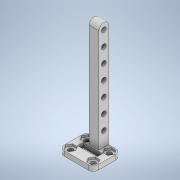
# Autodesk Inventor part: camera_stand
Saved by Autodesk Inventor 2020 (Build 240168000, 168)
## iProperties
Created: 2023-05-28
Part Number: camera_stand
Material: Generic
Document SubType Name: Modeling
Designer: denis
Density: 1 g/cm^3
Appearance: Default
Author: denis
Autodesk Inventor part; units mm, degrees
ref_plane "YZ Plane" through (0, 0, 0) normal (1, 0, 0) x (0, 1, 0)
ref_plane "XZ Plane" through (0, 0, 0) normal (0, 1, 0) x (-1, 0, 0)
ref_plane "XY Plane" through (0, 0, 0) normal (0, 0, 1) x (1, 0, 0)
sketch "Эскиз1" plane through (0, 0, 0) normal (1, 0, 0) x (0, 1, 0)
  line L0 (-2.5, 8.5) -> (0.5, 8.5)
  line L1 (0.5, 8.5) -> (0.5, -8.5)
  line L2 (0.5, -8.5) -> (-2.5, -8.5)
  line L3 (-2.5, -8.5) -> (-2.5, 8.5)
  line L4 (0.5, -8.5) -> (64.5, -8.5)
  line L5 (67.5, -5.5) -> (67.5, -5.5)
  line L6 (64.5, -2.5) -> (0.5, -2.5)
  line L7 (0.5, -2.5) -> (0.5, -8.5)
  circle A0 centre (9.5, -5.5) radius 1.5
  circle A1 centre (18.5, -5.5) radius 1.5
  circle A2 centre (27.5, -5.5) radius 1.5
  circle A3 centre (36.5, -5.5) radius 1.5
  circle A4 centre (45.5, -5.5) radius 1.5
  circle A5 centre (54.5, -5.5) radius 1.5
  circle A6 centre (63.5, -5.5) radius 1.5
  arc A7 (67.5, -5.5) -> (64.5, -2.5) centre (64.5, -5.5) ccw
  arc A8 (64.5, -8.5) -> (67.5, -5.5) centre (64.5, -5.5) ccw
  point P0 (0, 0)
  point P1 (67.5, -2.5)
  point P2 (67.5, -8.5)
  dimension "d0" = 3
  dimension "d1" = 17
  dimension "d2" = 67
  dimension "d3" = 6
  dimension "d4" = 3
  dimension "d5" = 9
  dimension "d6" = 3
  dimension "d7" = 9
  dimension "d8" = 3
  dimension "d9" = 9
  dimension "d10" = 3
  dimension "d11" = 9
  dimension "d12" = 3
  dimension "d13" = 9
  dimension "d14" = 3
  dimension "d15" = 9
  dimension "d16" = 3
  dimension "d17" = 9
  dimension "d18" = 3
  constraints: 16 end point, 9 centre point, 4 parallel, 4 point on circle, 4 point on line, 4 tangent, 2 horizontal, 2 perpendicular, 1 concentric
  measures "d0" distance of L1.end L2.end
  measures "d1" distance of L0.end L1.end
  measures "d2" distance of L6.end point (67.5, -2.5)
  measures "d3" distance of point (67.5, -2.5) point (67.5, -8.5)
  measures "d4" diameter of A0
  measures "d5" distance from line of L1 A0.centre
  measures "d6" diameter of A1
  measures "d7" distance of A0.centre A1.centre
  measures "d8" diameter of A2
  measures "d9" distance of A1.centre A2.centre
  measures "d10" diameter of A3
  measures "d11" distance of A2.centre A3.centre
  measures "d12" diameter of A4
  measures "d13" distance of A4.centre A3.centre
  measures "d14" diameter of A5
  measures "d15" distance of A4.centre A5.centre
  measures "d16" diameter of A6
  measures "d17" distance of A5.centre A6.centre
  measures "d18" radius of A7
extrude "Выдавливание1" add sketch "Эскиз1" along normal mid plane 21 contours L0 L1 L2 L3
extrude "Выдавливание2" add sketch "Эскиз1" along normal mid plane 6 contours L6 A7 A8 L4 L1
sketch "Эскиз3" plane through (-10.5, 0.5, 8.5) normal (0, 1, 0) x (1, 0, 0)
  line L0 (21, 0) -> (0, 0) projected
  line L1 (10.5, 0) -> (10.5, 17) construction
  line L2 (0, 17) -> (21, 17) projected
  line L3 (0, 17) -> (0, 0) construction
  line L4 (21, 0) -> (21, 17) construction
  line L5 (0, 0) -> (21, 17) construction
  line L6 (21, 0) -> (0, 17) construction
  line L7 (0, 8.5) -> (21, 8.5) construction
  circle A0 centre (3.5, 3.5) radius 1.5
  circle A1 centre (3.5, 13.5) radius 1.5
  circle A2 centre (17.5, 3.5) radius 1.5
  circle A3 centre (17.5, 13.5) radius 1.5
  line L8 (18, 0) -> (3, 0) construction
  line L9 (0, 3) -> (0, 14) construction
  line L10 (3, 17) -> (18, 17) construction
  line L11 (21, 14) -> (21, 3) construction
  line L12 (21, 0) -> (0, 17) construction
  line L13 (0, 0) -> (21, 17) construction
  arc A4 (3, 17) -> (0, 14) centre (3, 14) ccw
  arc A5 (0, 3) -> (3, 0) centre (3, 3) ccw
  arc A6 (18, 0) -> (21, 3) centre (18, 3) ccw
  arc A7 (21, 14) -> (18, 17) centre (18, 14) ccw
  line L14 (21, 0) -> (0, 0) construction
  line L15 (0, 0) -> (0, 17) construction
  line L16 (0, 17) -> (21, 17) construction
  line L17 (21, 17) -> (21, 0) construction
  line L18 (21, 0) -> (0, 17) construction
  line L19 (0, 0) -> (21, 17) construction
  line L20 (3, 0) -> (0, 0)
  line L21 (0, 0) -> (0, 3)
  line L22 (0, 14) -> (0, 17)
  line L23 (3, 17) -> (0, 17)
  line L24 (18, 17) -> (21, 17)
  line L25 (21, 17) -> (21, 14)
  line L26 (21, 3) -> (21, 0)
  line L27 (21, 0) -> (18, 0)
  line L28 (16.5, 6.75) -> (4.5, 6.75)
  line L29 (4.5, 6.75) -> (4.5, 10.25)
  line L30 (4.5, 10.25) -> (16.5, 10.25)
  line L31 (16.5, 10.25) -> (16.5, 6.75)
  line L32 (16.5, 6.75) -> (4.5, 10.25) construction
  line L33 (4.5, 6.75) -> (16.5, 10.25) construction
  line L34 (17.5, 3.5) -> (17.5, 0.65) construction
  line L35 (17.5, 0.65) -> (17.5, 6.35) construction
  line L36 (17.5, 3.5) -> (14.4, 3.5) construction
  line L37 (14.4, 3.5) -> (20.6, 3.5) construction
  line L38 (15.95, 0.8153) -> (14.4, 3.5)
  line L39 (14.4, 3.5) -> (15.95, 6.1847)
  line L40 (15.95, 6.1847) -> (19.05, 6.1847)
  line L41 (19.05, 6.1847) -> (20.6, 3.5)
  line L42 (20.6, 3.5) -> (19.05, 0.8153)
  line L43 (19.05, 0.8153) -> (15.95, 0.8153)
  line L44 (15.95, 10.8153) -> (14.4, 13.5)
  line L45 (15.95, 16.1847) -> (14.4, 13.5)
  line L46 (15.95, 10.8153) -> (19.05, 10.8153)
  line L47 (19.05, 10.8153) -> (20.6, 13.5)
  line L48 (20.6, 13.5) -> (19.05, 16.1847)
  line L49 (19.05, 16.1847) -> (15.95, 16.1847)
  line L50 (1.95, 0.8153) -> (0.4, 3.5)
  line L51 (0.4, 3.5) -> (1.95, 6.1847)
  line L52 (1.95, 6.1847) -> (5.05, 6.1847)
  line L53 (5.05, 6.1847) -> (6.6, 3.5)
  line L54 (6.6, 3.5) -> (5.05, 0.8153)
  line L55 (5.05, 0.8153) -> (1.95, 0.8153)
  line L56 (1.95, 10.8153) -> (0.4, 13.5)
  line L57 (0.4, 13.5) -> (1.95, 16.1847)
  line L58 (1.95, 16.1847) -> (5.05, 16.1847)
  line L59 (5.05, 16.1847) -> (6.6, 13.5)
  line L60 (6.6, 13.5) -> (5.05, 10.8153)
  line L61 (5.05, 10.8153) -> (1.95, 10.8153)
  point P0 (10.5, 8.5)
  point P1 (3, 0)
  dimension "d23" = 3
  dimension "d24" = 10
  dimension "d25" = 14
  dimension "d26" = 3
  dimension "d29" = 12
  dimension "d30" = 3.5
  constraints: 116 end point, 15 parallel, 11 point on line, 11 tangent, 10 midpoint, 9 horizontal, 8 centre point, 8 point on circle, 5 coincident, 5 collinear, 5 perpendicular, 4 equal length, 3 equal radius, 3 symmetric about line, 1 vertical, 3 other
  measures "d23" diameter of A0
  measures "d24" distance of A1.centre A0.centre
  measures "d25" distance of A0.centre L34.start
  measures "d26" radius of A4
  measures "d29" distance of L29.end L30.end
  measures "d30" distance of L28.end L29.end
extrude "Выдавливание3" cut sketch "Эскиз3" against normal blind 6 contours L0 L21 A5 | L0 A6 L26 | L2 L25 A7 | L2 A4 L22 | A0 | A1 | A2 | A3 | L28 L29 L30 L31
extrude "Выдавливание4" cut sketch "Эскиз3" against normal blind 1.2 contours L38 L39 L40 L41 L42 L43 | L44 L45 L49 L48 L47 L46 | L50 L51 L52 L53 L54 L55 | L56 L57 L58 L59 L60 L61
